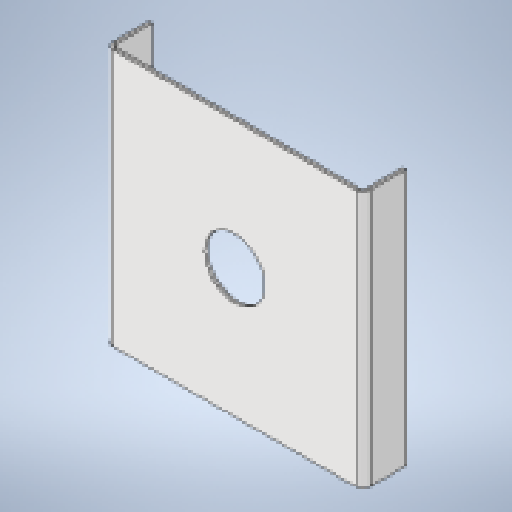
# Autodesk Inventor part: FL3.6.2  Motor pillar
Saved by Autodesk Inventor 2025.1 (Build 291241020, 241B)
## iProperties
Created: 2023-03-28
Part Number: FL3.6.2  Motor pillar
Material: Stainless Steel
Document SubType Name: Sheet Metal
Designer: user
Density: 8 g/cm^3
Sheet Metal Rule: Default_mm
Appearance: Default
Flat Pattern Width: 22.3048 cm
Flat Pattern Length: 15 cm
Flat Pattern Area: 334.572 cm^2
Sheet Metal Width: 223.048 mm
Sheet Metal Length: 150.000 mm
Sheet Metal Area: 33457.168 mm^2
Stock Number: bend
Description: bend
Author: user
Autodesk Inventor part; units mm, degrees
ref_plane "YZ Plane" through (0, 0, 0) normal (1, 0, 0) x (0, 1, 0)
ref_plane "XZ Plane" through (0, 0, 0) normal (0, 1, 0) x (-1, 0, 0)
ref_plane "XY Plane" through (0, 0, 0) normal (0, 0, 1) x (1, 0, 0)
sketch "Sketch1" plane through (0, 0, 0) normal (0, 0, 1) x (1, 0, 0)
  line L0 (75, 0) -> (-75, 0)
  line L1 (-75, 0) -> (-75, 150)
  line L2 (-75, 150) -> (75, 150)
  line L3 (75, 150) -> (75, 0)
  point P0 (0, 0)
  point P1 (0, 0)
  dimension "d1" = 150
  dimension "d2" = 150
  constraints: 8 end point, 2 parallel, 1 coincident, 1 horizontal, 1 midpoint, 1 perpendicular
  measures "d1" distance of L2.end L0.start
  measures "d2" distance of L1.end L2.end
extrude "Plate1" add sketch "Sketch1" along normal blind 2
sketch "Sketch2" plane through (0, 0, 0) normal (0, 0, 1) x (1, 0, 0)
  line L0 (-75, 0) -> (-75, 150) projected
  line L1 (75, 0) -> (-75, 0) projected
  line L2 (75, 150) -> (75, 0) projected
  line L3 (-75, 150) -> (75, 150) projected
  circle A0 centre (0, 75) radius 17.5
  line L4 (45, 40) -> (-45, 40) construction
  line L5 (-45, 40) -> (-45, 110) construction
  line L6 (-45, 110) -> (45, 110) construction
  line L7 (45, 110) -> (45, 40) construction
  line L8 (45, 40) -> (-45, 110) construction
  line L9 (-45, 40) -> (45, 110) construction
  circle A1 centre (-45, 40) radius 4
  circle A2 centre (45, 40) radius 4
  circle A3 centre (45, 110) radius 4
  circle A4 centre (-45, 110) radius 4
  point P0 (0, 0)
  point P1 (0, 0)
  point P2 (75, 75)
  dimension "d3" = 35
  dimension "d4" = 90
  dimension "d5" = 70
  dimension "d7" = 8
  constraints: 12 end point, 5 centre point, 4 coincident, 4 midpoint, 3 equal radius, 2 parallel, 1 horizontal, 1 horizontal alignment, 1 perpendicular, 1 vertical alignment
  measures "d3" diameter of A0
  measures "d4" distance of L4.start L4.end
  measures "d5" distance of L4.end L5.end
  measures "d7" diameter of A1
extrude "Extrusion1" cut sketch "Sketch2" along normal through all contours A1 | A2 | A3 | A4
sketch "Sketch3" plane through (-73, 150, 2) normal (-1, 0, 0) x (0, -1, 0)
  line L0 (150, 0) -> (0, 0)
  line L1 (0, 0) -> (0, -40)
  line L2 (0, -40) -> (150, -40)
  line L3 (150, -40) -> (150, 0)
  constraints: 6 end point, 1 horizontal, 1 perpendicular, 1 vertical
edge flange "Flange1" height 40 angle 90 thickness 2 bend radius 2 thickness toward (-1, 0, 0) relief straight relief width 2 relief depth 1 corner gap 2 corner form 0 edges at (-75, 75, 0) (75, 75, 0) wall of the first edge with corners at (-73, 0, 2) (-73, 150, 2) (-73, 150, -38) (-73, 0, -38)
bend "Bend1"
corner "Corner1"
sketch "Sketch4" plane through (0, 0, 0) normal (0, 0, 1) x (1, 0, 0)
  circle A0 centre (0, 75) radius 17.5 projected
  line L0 (0, 125) -> (0, 105) construction
  line L1 (-3, 125) -> (-3, 105)
  line L2 (3, 105) -> (3, 125)
  arc A1 (3, 125) -> (-3, 125) centre (0, 125) ccw
  arc A2 (-3, 105) -> (3, 105) centre (0, 105) ccw
  arc A3 (34.641, 95) -> (20, 109.641) centre (0, 75) ccw construction
  arc A4 (37.2391, 96.5) -> (21.5, 112.2391) centre (0, 75) ccw
  arc A5 (32.0429, 93.5) -> (18.5, 107.0429) centre (0, 75) ccw
  arc A6 (32.0429, 93.5) -> (37.2391, 96.5) centre (34.641, 95) ccw
  arc A7 (21.5, 112.2391) -> (18.5, 107.0429) centre (20, 109.641) ccw
  line L3 (0, 75) -> (20, 109.641) construction
  line L4 (0, 75) -> (40, 75) construction
  line L5 (0, 75) -> (34.641, 95) construction
  point P0 (0, 0)
  point P1 (0, 115)
  dimension "d20" = 20
  dimension "d21" = 6
  dimension "d22" = 30
  dimension "d23" = 60
  dimension "d24" = 30
  dimension "d25" = 6
  dimension "d26" = 40
  constraints: 14 end point, 14 point on circle, 8 tangent, 7 centre point, 1 coincident, 1 equal length, 1 horizontal, 1 midpoint, 1 parallel, 1 vertical, 1 vertical alignment
  measures "d20" distance of L0.start L0.end
  measures "d21" diameter of A2
  measures "d22" distance of A0.centre L0.end
  measures "d23" angle of L4 L3
  measures "d24" angle of L5 L3
  measures "d25" diameter of A6
  measures "d26" radius of A3
extrude "Extrusion2" [suppressed]
pattern_circular "Circular Pattern1" [suppressed]
equation "\"d1\" = d2"
equation "\"d0\" = Thickness"
equation "\"d10\" = BendReliefWidth"
equation "\"d11\" = BendReliefDepth"
equation "\"d12\" = MinimumRemnant"
equation "\"d13\" = TransitionRadius"
equation "\"d16\" = BendRadius"
equation "\"d17\" = CornerReliefSize"
equation "\"d18\" = GapSize"
equation "\"d19\" = JacobiRadiusSize"
equation "\"BendRadius\" = Thickness"
equation "\"BendReliefWidth\" = Thickness"
equation "\"BendReliefDepth\" = 0.5 * Thickness"
equation "\"CornerReliefSize\" = 4 * Thickness"
equation "\"MinimumRemnant\" = 2 * Thickness"
equation "\"TransitionRadius\" = BendRadius"
equation "\"JacobiRadiusSize\" = BendRadius"
equation "\"GapSize\" = Thickness"
equation "\"Thickness\" = 2"
body "Solid1"
